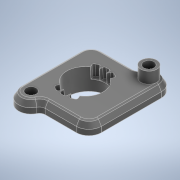
# Autodesk Inventor part: coil_pack_adapter_plate
Saved by Autodesk Inventor 2021 (Build 250183000, 183)
## iProperties
Created: 2021-09-22
Part Number: coil_pack_adapter_plate
Material: Generic
Document SubType Name: Modeling
Designer: Andrew
Density: 1 g/cm^3
Appearance: Default
Author: Andrew
Autodesk Inventor part; units mm, degrees
ref_plane "YZ Plane" through (0, 0, 0) normal (1, 0, 0) x (0, 1, 0)
ref_plane "XZ Plane" through (0, 0, 0) normal (0, 1, 0) x (-1, 0, 0)
sketch "Body_sketch" plane through (0, 0, 0) normal (0, 1, 0) x (-1, 0, 0)
  line L0 (32, 0) -> (-32, 0)
  line L1 (-32, 0) -> (-32, -31)
  line L2 (32, -22) -> (32, 0)
  circle A0 centre (-21, -31) radius 4.55
  arc A1 (-32, -31) -> (-11.1086, -35.8125) centre (-21, -31) ccw
  line L3 (-6.6125, -33) -> (21, -33)
  arc A2 (-6.6125, -33) -> (-11.1086, -35.8125) centre (-6.6125, -38) ccw
  arc A3 (21, -33) -> (32, -22) centre (21, -22) ccw
  line L4 (27.7, 0) -> (27.7, -22)
  line L5 (30.7, 0) -> (30.7, -22)
  line L6 (21, -28.7) -> (-6.6125, -28.7)
  line L7 (21, -31.7) -> (-6.6125, -31.7)
  arc A4 (21, -31.7) -> (30.7, -22) centre (21, -22) ccw
  arc A5 (21, -28.7) -> (27.7, -22) centre (21, -22) ccw
  arc A6 (-6.6125, -28.7) -> (-14.9752, -33.9312) centre (-6.6125, -38) ccw
  arc A7 (-6.6125, -31.7) -> (-12.2776, -35.2437) centre (-6.6125, -38) ccw
  arc A8 (-27.7, -31) -> (-14.9752, -33.9312) centre (-21, -31) ccw
  arc A9 (-30.7, -31) -> (-12.2776, -35.2437) centre (-21, -31) ccw
  line L8 (-30.7, -31) -> (-30.7, 0)
  line L9 (-27.7, -31) -> (-27.7, 0)
  line L10 (-29.9, 0) -> (-29.9, -1)
  line L11 (-29.9, -1) -> (-30.7, -1)
  line L12 (-27.7, -29) -> (-28.5, -29)
  line L13 (-28.5, -29) -> (-28.5, -31)
  line L14 (-28.5, -31) -> (-27.7, -31)
  line L15 (-4.6125, -31.7) -> (-4.6125, -30.9)
  line L16 (-4.6125, -30.9) -> (-6.6125, -30.9)
  line L17 (-6.6125, -30.9) -> (-6.6125, -31.7)
  line L18 (19, -28.7) -> (19, -29.5)
  line L19 (19, -29.5) -> (21, -29.5)
  line L20 (21, -29.5) -> (21, -28.7)
  line L21 (30.7, -20) -> (29.9, -20)
  line L22 (29.9, -20) -> (29.9, -22)
  line L23 (29.9, -22) -> (30.7, -22)
  line L24 (27.7, -1) -> (28.5, -1)
  line L25 (28.5, -1) -> (28.5, 0)
  line L26 (27.7, -22) -> (28.5, -22)
  line L27 (28.5, -22) -> (28.5, -20)
  line L28 (28.5, -20) -> (27.7, -20)
  line L29 (21, -31.7) -> (21, -30.9)
  line L30 (21, -30.9) -> (19, -30.9)
  line L31 (19, -30.9) -> (19, -31.7)
  line L32 (-6.6125, -28.7) -> (-6.6125, -29.5)
  line L33 (-6.6125, -29.5) -> (-4.6125, -29.5)
  line L34 (-4.6125, -29.5) -> (-4.6125, -28.7)
  line L35 (-30.7, -31) -> (-29.9, -31)
  line L36 (-29.9, -31) -> (-29.9, -29)
  line L37 (-29.9, -29) -> (-30.7, -29)
  line L38 (-26.7, 0) -> (-26.7, -27.4786)
  arc A10 (-14.3016, -31.1467) -> (-26.7, -27.4786) centre (-21, -31) ccw
  line L39 (-3.6213, -1.5) -> (-26.7, -24.5787)
  line L40 (-1.5, -3.6213) -> (-22.3075, -24.4288)
  line L41 (-1.5, -3.6213) -> (-1.5, -28.7)
  line L42 (1.5, -28.7) -> (1.5, -3.6213)
  line L43 (1.5, -3.6213) -> (24.4307, -26.552)
  line L44 (26.2768, -24.1554) -> (3.6213, -1.5)
  line L45 (-3.6213, -1.5) -> (-26.7, -1.5)
  line L46 (0, 0) -> (-27.7, -27.7) construction
  line L47 (0, 0) -> (0, -28.7) construction
  line L48 (0, 0) -> (27.7, -27.7) construction
  arc A11 (-6.6125, -27.7) -> (-14.3016, -31.1467) centre (-6.6125, -38) ccw
  line L49 (-6.6125, -27.7) -> (21, -27.7)
  arc A12 (21, -27.7) -> (26.7, -22) centre (21, -22) ccw
  line L50 (26.7, -22) -> (26.7, 0)
  line L51 (3.6213, -1.5) -> (26.7, -1.5)
  line L52 (-28.2, 0) -> (-28.2, -31)
  line L53 (-30.2, 0) -> (-30.2, -31)
  line L54 (-6.6125, -29.2) -> (21, -29.2)
  line L55 (21, -31.2) -> (-6.6125, -31.2)
  line L56 (30.2, 0) -> (30.2, -22)
  line L57 (28.2, 0) -> (28.2, -22)
  arc A13 (21, -29.2) -> (28.2, -22) centre (21, -22) ccw
  arc A14 (21, -31.2) -> (30.2, -22) centre (21, -22) ccw
  arc A15 (-6.6125, -29.2) -> (-14.5256, -34.15) centre (-6.6125, -38) ccw
  arc A16 (-6.6125, -31.2) -> (-12.7272, -35.025) centre (-6.6125, -38) ccw
  arc A17 (-28.2, -31) -> (-14.5256, -34.15) centre (-21, -31) ccw
  arc A18 (-30.2, -31) -> (-12.7272, -35.025) centre (-21, -31) ccw
  point P0 (-10.1833, -33)
  point P1 (1.5, -27.7)
  point P2 (-1.5, -27.7)
  dimension "d2" = 32
  dimension "d3" = 31
  dimension "d4" = 9.1
  dimension "d5" = 21
  dimension "d6" = 33
  dimension "d7" = 5
  dimension "d8" = 11
  dimension "d9" = 3
  dimension "d10" = 1.3
  dimension "d21" = 0.8
  dimension "d22" = 0.8
  dimension "d23" = 0.8
  dimension "d24" = 0.8
  dimension "d25" = 0.8
  dimension "d26" = 0.8
  dimension "d27" = 2
  dimension "d28" = 2
  dimension "d29" = 2
  dimension "d30" = 2
  dimension "d31" = 1
  dimension "d32" = 1
  dimension "d34" = 0.8
  dimension "d35" = 0.8
  dimension "d36" = 0.8
  dimension "d37" = 0.8
  dimension "d170" = 1
  dimension "d173" = 3
  dimension "d174" = 45
  dimension "d175" = 45
  dimension "d176" = 3
  dimension "d177" = 3
  dimension "d178" = 1
  dimension "d179" = 1.5
  dimension "d195" = 0.5
  dimension "d196" = 2
  constraints: 114 end point, 40 point on circle, 29 tangent, 22 perpendicular, 19 centre point, 19 point on line, 17 vertical, 15 concentric, 10 horizontal, 5 collinear, 3 parallel, 2 coincident, 19 other
  measures "d2" distance from line of point (0, 0) L1
  measures "d3" vertical distance of point (0, 0) A0.centre
  measures "d4" diameter of A0
  measures "d5" horizontal distance of A0.centre point (0, 0)
  measures "d6" distance from line of point (0, 0) L3
  measures "d7" radius of A2
  measures "d8" radius of A3
  measures "d9" distance between parallel lines of L5 L4
  measures "d10" distance between parallel lines of L2 L5
  measures "d21" distance between parallel lines of L7 L16
  measures "d22" distance of L10.end L11.end
  measures "d23" distance of L12.start L12.end
  measures "d24" distance of L18.start L18.end
  measures "d25" distance of L5.end L22.end
  measures "d26" distance of L24.start L24.end
  measures "d27" distance of L21.end L22.end
  measures "d28" distance of L18.end L19.end
  measures "d29" distance of L15.end L16.end
  measures "d30" distance of L12.end L13.end
  measures "d31" distance of L10.start L10.end
  measures "d32" distance of L24.end L25.end
  measures "d34" distance of L36.end L37.end
  measures "d35" distance of L6.end L32.end
  measures "d36" distance of L30.end L31.end
  measures "d37" distance of L4.end L26.end
  measures "d170" distance between parallel lines of L38 L9
  measures "d173" distance between parallel lines of L40 L39
  measures "d174" angle of L47 L46
  measures "d175" angle of L48 L47
  measures "d176" distance between parallel lines of L42 L41
  measures "d177" distance between parallel lines of L44 L43
  measures "d178" distance between parallel lines of L4 L50
  measures "d179" distance of the line from the sketch origin of L45
  measures "d195" distance between parallel lines of L5 L56
  measures "d196" distance between parallel lines of L56 L57
sketch "reservoir offset sketch" plane through (0, 0, 0) normal (0, 1, 0) x (-1, 0, 0)
  circle A0 centre (-21, -31) radius 4.55 projected
  arc A1 (-32, -31) -> (-11.1086, -35.8125) centre (-21, -31) ccw projected
  circle A2 centre (-21, -31) radius 7
  point P0 (0, 0)
  dimension "d218" = 14
  constraints: 1 centre point, 1 coincident
  measures "d218" diameter of A2
extrude "Extrusion1" add sketch "Body_sketch" along normal blind 10
extrude "Extrusion14" add sketch "reservoir offset sketch" along normal blind 20 separate body
chamfer "Chamfer1" distance 3 angle 60 6 edges at (32, 10, -15.5) (23.4693, 10, -41.7193) (9.2642, 10, -33.761) (-7.1937, 10, -33) (-28.7782, 10, -29.7782) (-32, 10, -11) measured on face at (-28.4246, 10, -29.4246) measured on face at (23.357, 10, -41.232) measured on face at (-31.5, 10, -11) measured on face at (31.5, 10, -15.5) measured on face at (9.5293, 10, -33.3371) measured on face at (-7.1937, 10, -32.5)
chamfer "Chamfer2" distance 1 angle 45 6 edges at (29, 10, -15.5) (22.7958, 10, -38.7958) (10.8551, 10, -31.2177) (-7.1937, 10, -30) (-26.6569, 10, -27.6569) (-29, 10, -11)
combine bodies "Combine14" operation type subtract main body 2 bodies to subtract 1 keep tools yes
extrude "Extrusion2" cut sketch "Body_sketch" along normal blind 2 contours L5 L21 L56 L0 | L56 L21 L22 L23 A14 L29 L30 L31 L55 L15 L16 L17 A16 A18 L35 L36 L37 L53 L11 L10 L0 L52 L12 L13 L14 A17 A15 L32 L33 L34 L54 L18 L19 L20 A13 L26 L27 L28 L57 L24 L25 | L5 L23 L56 L21 | L25 L24 L57 L0 | L56 L23 L22 L21 | A4 L29 A14 L23 | L57 L24 L4 L0 | L7 L31 L55 L29 | L57 L28 L4 L24 | L55 L31 L30 L29 | L7 L15 L55 L31 | L57 L26 L4 L28 | L28 L27 L26 L57 | L7 L17 L55 L15 | A13 L20 A5 L26 | L55 L17 L16 L15 | A7 A9 L35 A18 A16 L17 | L0 L53 L11 L8 | L9 L12 L52 L0 | L54 L18 L6 L20 | L20 L19 L18 L54 | L0 L10 L11 L53 | L11 L53 L37 L8 | L9 L14 L52 L12 | L54 L34 L6 L18 | L8 L37 L53 L35 | L52 L14 L13 L12 | A8 A6 L32 A15 A17 L14 | L54 L32 L6 L34 | L34 L33 L32 L54 | L53 L37 L36 L35 bodies 1
mirror "Mirror1" about plane through (0, 0, 0) normal (0, 0, 1) bodies 1 separate body
mirror "Mirror2" about plane through (0, 0, 0) normal (1, 0, 0) remove original yes bodies 3
extrude "Extrusion3" add sketch "Body_sketch" along normal up to surface (2 mm away) separate body contours L7 L31 L55 L29 | L55 L31 L30 L29 | L57 L26 L4 L28 | L28 L27 L26 L57 | L8 L37 L53 L35 | L54 L32 L6 L34 | L34 L33 L32 L54 | L53 L37 L36 L35
mirror "Mirror3" about plane through (0, 0, 0) normal (0, 0, 1) remove original yes bodies 4
mirror "Mirror5" about plane through (0, 0, 0) normal (1, 0, 0) remove original yes bodies 4
extrude "Extrusion4" add sketch "Body_sketch" along normal up to surface (2 mm away) separate body contours L5 L23 L56 L21 | L56 L23 L22 L21 | L7 L17 L55 L15 | L55 L17 L16 L15 | L54 L18 L6 L20 | L20 L19 L18 L54 | L9 L14 L52 L12 | L52 L14 L13 L12
extrude "Extrusion5" add sketch "Body_sketch" along normal up to surface (2 mm away) separate body contours L25 L24 L57 L0 | L57 L24 L4 L0 | L0 L53 L11 L8 | L0 L10 L11 L53
mirror "Mirror6" about plane through (0, 0, 0) normal (0, 0, 1) bodies 6
combine bodies "Combine3" operation type add bodies to combine 1 3
combine bodies "Combine4" operation type add bodies to combine 6 5
combine bodies "Combine5" operation type add bodies to combine 6 4
combine bodies "Combine6" operation type add bodies to combine 1 6
extrude "Extrusion11" add sketch "Body_sketch" along normal blind 7 separate body contours L50 A12 L44 L51 | L45 L39 L38 | A12 L49 L42 L43 | L40 L41 L49 A11 A10
fillet "Fillet1" radius 1.5 9 edges at (26.7, 3.5, -24.5787) (22.3075, 3.5, -24.4288) (14.3016, 3.5, -31.1467) (1.5, 3.5, -27.7) (-1.5, 3.5, -27.7) (-24.4307, 3.5, -26.552) (-26.2768, 3.5, -24.1554) (26.7, 3.5, -1.5) (-26.7, 3.5, -1.5)
mirror "Mirror11" about plane through (0, 0, 0) normal (0, 0, 1) bodies 7 separate body
mirror "Mirror12" about plane through (0, 0, 0) normal (1, 0, 0) remove original yes bodies 8
combine bodies "Combine8" operation type add bodies to combine 7 8
combine bodies "Combine9" operation type subtract main body 1 bodies to subtract 7
sketch "Ignition Coil Positioning" plane through (0, 0, 0) normal (0, 0, 1) x (1, 0, 0)
  line L0 (-25, 13.5) -> (-24.8039, 11.0077)
  line L1 (-24.8039, 11.0077) -> (15.5713, 14.1853)
  line L2 (15.5713, 14.1853) -> (15.3752, 16.6776)
  line L3 (15.3752, 16.6776) -> (-25, 13.5)
  line L4 (-32, 10) -> (32, 10)
  line L5 (32, 10) -> (32, 14.1853)
  line L6 (32, 14.1853) -> (-32, 14.1853)
  line L7 (-32, 14.1853) -> (-32, 10)
  line L8 (-4.8124, 15.0888) -> (-3.6249, 0) construction
  line L9 (0, 19.5902) -> (0, -3.265) projected
  point P0 (0, 0)
  point P1 (-32, 0)
  point P2 (-32, 0)
  point P3 (32, 0)
  point P4 (32, 0)
  point P5 (32, 0)
  point P6 (-16.2924, 14.1853)
  dimension "d127" = 40.5
  dimension "d129" = 2.5
  dimension "d185" = 10
  dimension "d208" = 7
  dimension "d213" = 13.5
  dimension "d221" = 4.5
  dimension "d222" = 14.1853
  constraints: 18 end point, 4 parallel, 3 perpendicular, 3 point on line, 1 horizontal, 1 horizontal alignment, 1 midpoint
  measures "d127" distance of L2.end L0.start
  measures "d129" distance of L1.end L2.end
  measures "d185" distance from line of point (0, 0) L4
  measures "d208" horizontal distance of point (-32, 0) L0.start
  measures "d213" vertical distance of point (-32, 0) L0.start
  measures "d221" angle of L9 L8
  measures "d222" vertical distance of point (0, 0) L1.end
ref_plane "Work Plane3" through (-24.8039, 11.0077, 0) normal (0.0784591, -0.9969173, 0) x (0.9969173, 0.0784591, 0)
sketch "Ignition Coil Mount" plane through (-24.8039, 11.0077, 0) normal (0.0784591, -0.9969173, 0) x (0.9969173, 0.0784591, 0)
  line L0 (0, 0) -> (40.5, 0) construction
  line L1 (20.25, -20) -> (21.75, -20)
  line L2 (23.25, -18.5) -> (23.25, -15.7162)
  line L3 (23.4927, -15.668) -> (24.558, -18.2398)
  line L4 (26.5178, -19.0516) -> (29.2895, -17.9036)
  line L5 (30.1013, -15.9437) -> (29.036, -13.3719)
  line L6 (20.25, 0) -> (27.9037, -18.4776) construction
  line L7 (20.25, 0) -> (20.25, -20)
  line L8 (20.25, -21.5) -> (23.5321, -21.5)
  line L9 (25.4455, -21.1194) -> (29.8635, -19.2894)
  line L10 (31.4871, -15.3697) -> (31.7086, -15.9044)
  arc A0 (32.3978, -12.5969) -> (37.75, 0) centre (20.25, 0) ccw
  arc A1 (20.25, -16) -> (36.25, 0) centre (20.25, 0) ccw
  line L11 (20.25, -20) -> (20.25, -21.5)
  arc A2 (23.5321, -21.5) -> (25.4455, -21.1194) centre (23.5321, -16.5) ccw
  arc A3 (32.3978, -12.5969) -> (31.7086, -15.9044) centre (34.4802, -14.7564) ccw
  line L12 (20.25, 0) -> (37.75, 0)
  arc A4 (21.75, -20) -> (23.25, -18.5) centre (21.75, -18.5) ccw
  arc A5 (24.558, -18.2398) -> (26.5178, -19.0516) centre (25.9438, -17.6658) ccw
  arc A6 (29.2895, -17.9036) -> (30.1013, -15.9437) centre (28.7155, -16.5177) ccw
  arc A7 (29.8635, -19.2894) -> (31.4871, -15.3697) centre (28.7155, -16.5177) ccw
  point P0 (23.8637, 0)
  point P1 (23.25, -20)
  point P2 (32.6352, -18.1413)
  point P3 (30.8792, -13.9021)
  dimension "d134" = 1.5
  dimension "d143" = 1.5
  dimension "d145" = 20
  dimension "d146" = 20
  dimension "d148" = 22.5
  dimension "d150" = 16
  dimension "d151" = 3
  dimension "d152" = 3
  dimension "d154" = 1.5
  dimension "d155" = 5
  dimension "d156" = 1.5
  dimension "d157" = 3
  dimension "d190" = 1.5
  dimension "d191" = 1.5
  dimension "d192" = 1.5
  dimension "d193" = 3
  constraints: 25 end point, 20 point on circle, 12 tangent, 8 centre point, 8 point on line, 2 midpoint, 2 parallel, 2 perpendicular, 2 vertical, 1 coincident, 1 collinear, 1 other
  measures "d134" distance between parallel lines of L1 L8
  measures "d143" distance between parallel lines of L9 L4
  measures "d145" distance of L1.start L6.start
  measures "d146" distance of L6.start L6.end
  measures "d148" angle of L6 L7
  measures "d150" radius of A1
  measures "d151" distance between parallel lines of L2 L7
  measures "d152" distance between parallel lines of L5 L6
  measures "d154" radial gap between concentric circles of A1 A0
  measures "d155" radius of A2
  measures "d156" distance between parallel lines of L5 L10
  measures "d157" radius of A3
  measures "d190" radius of A4
  measures "d191" radius of A5
  measures "d192" radius of A6
  measures "d193" radius of A7
extrude "Extrusion9" add sketch "Ignition Coil Mount" along normal mid plane 50 separate body
mirror "Mirror7" about plane through (12.8298, 13.9695, 0) normal (0, 0, 1) bodies 9
mirror "Mirror8" about plane through (-4.6163, 12.5965, 0) normal (-0.9969173, -0.0784591, 0) bodies 9
combine bodies "Combine7" operation type subtract main body 1 bodies to subtract 9
extrude "Extrusion6" add sketch "Ignition Coil Mount" along normal blind 20 separate body contours L7 A1 L2 A4 L1 | L1 A4 L2 A1 L3 A5 L4 A6 L5 L12 A0 A3 L10 A7 L9 A2 L8 L11 | A1 L5 A6 L4 A5 L3
extrude "Extrusion7" cut sketch "Ignition Coil Mount" along normal blind 11 contours L7 A1 L2 A4 L1 | L7 L12 A1 | A1 L5 A6 L4 A5 L3 bodies 10
mirror "Mirror9" about plane through (12.8298, 13.9695, 0) normal (0, 0, 1) bodies 10
mirror "Mirror10" about plane through (-4.6163, 12.5965, -16) normal (-0.9969173, -0.0784591, 0) bodies 10
extrude "Extrusion12" cut sketch "Ignition Coil Positioning" against normal through all both and the other way through all contours L0 L1 L9 L4 L7 L6 L3 | L1 L6 L5 L4 L9 bodies 10
combine bodies "Combine10" operation type add bodies to combine 1 10
fillet "Fillet2" radius 1.5 12 edges at (13.5891, 3.5, 1.5) (11.1417, 3.505, 9.0204) (11.1417, 3.505, -9.0204) (13.5891, 3.5, -1.5) (9.3533, 3.5014, -11.4747) (1.5, 4.0503, -21.0235) (-15.5029, 3.5383, -13.3816) (-21.3899, 3.5, -1.5) (-21.3899, 3.5, 1.5) (-15.5029, 3.5383, 13.3816) (9.3533, 3.5014, 11.4747) (1.5, 4.0503, 21.0235)
extrude "Extrusion13" add sketch "Body_sketch" along normal blind 2 and the other way blind 1 separate body contours L56 L21 L22 L23 A14 L29 L30 L31 L55 L15 L16 L17 A16 A18 L35 L36 L37 L53 L11 L10 L0 L52 L12 L13 L14 A17 A15 L32 L33 L34 L54 L18 L19 L20 A13 L26 L27 L28 L57 L24 L25 | L25 L24 L57 L0 | L56 L23 L22 L21 | L55 L31 L30 L29 | L28 L27 L26 L57 | L55 L17 L16 L15 | L20 L19 L18 L54 | L0 L10 L11 L53 | L52 L14 L13 L12 | L34 L33 L32 L54 | L53 L37 L36 L35
mirror "Mirror13" about plane through (0, 0, 0) normal (0, 0, 1) bodies 11 separate body
mirror "Mirror14" about plane through (0, 0, 0) normal (1, 0, 0) remove original yes bodies 12
combine bodies "Combine11" operation type add bodies to combine 11 12
equation "\"d21\" = d23"
equation "\"d22\" = d23"
equation "\"d24\" = d23"
equation "\"d25\" = d23"
equation "\"d26\" = d23"
equation "\"d27\" = d30"
equation "\"d28\" = d30"
equation "\"d29\" = d30"
equation "\"d31\" = 0.5 * d30"
equation "\"d32\" = d31"
equation "\"d34\" = d23"
equation "\"d35\" = d23"
equation "\"d36\" = d23"
equation "\"d37\" = d23"
equation "\"d146\" = d145"
equation "\"d152\" = d151"
